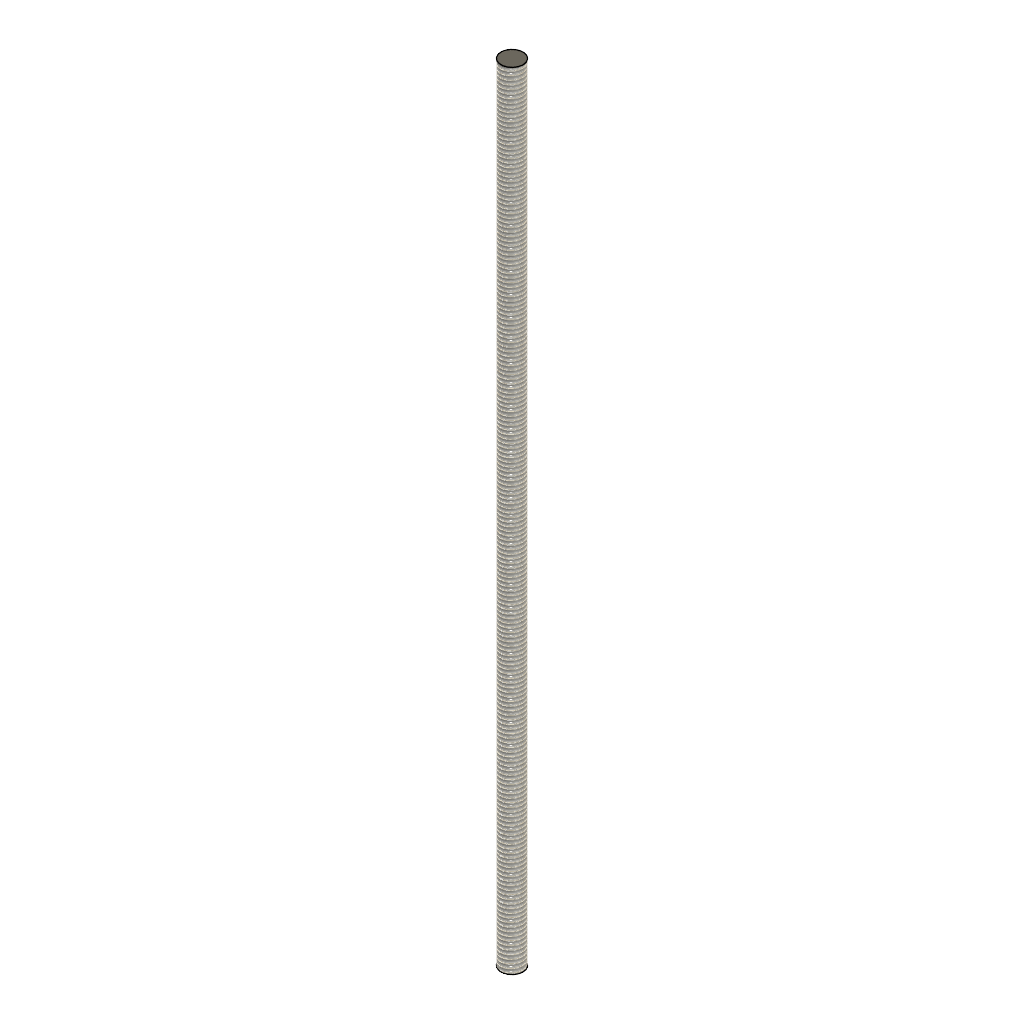
ROBOT_BALANCIN (Autodesk Fusion 360 archive; units mm, degrees)
design "M4_SIN_FIN"
Autodesk Fusion 360 part; units mm, degrees
(part 1 of 2)
sketch "Boceto1" plane through (0, 0, 0) normal (0, 0, 1) x (1, 0, 0)
  circle A0 centre (0, 0) radius 2
  dimension "d1" = 4
  constraint coincident A0.centre origin
  measures "d1" diameter of A0
extrude "Extruir1" add sketch "Boceto1" along normal blind 138
thread "Rosca1" "ISO Metric profile 4.0 M4x0.7 M4x0.7 6g" major diameter 3.908 minor diameter 3.111 pitch 0.7 angle 60 resizes the face on face at (1.9975, -0.0997, 92)
equation "d2 = 150 mm - 12 mm"

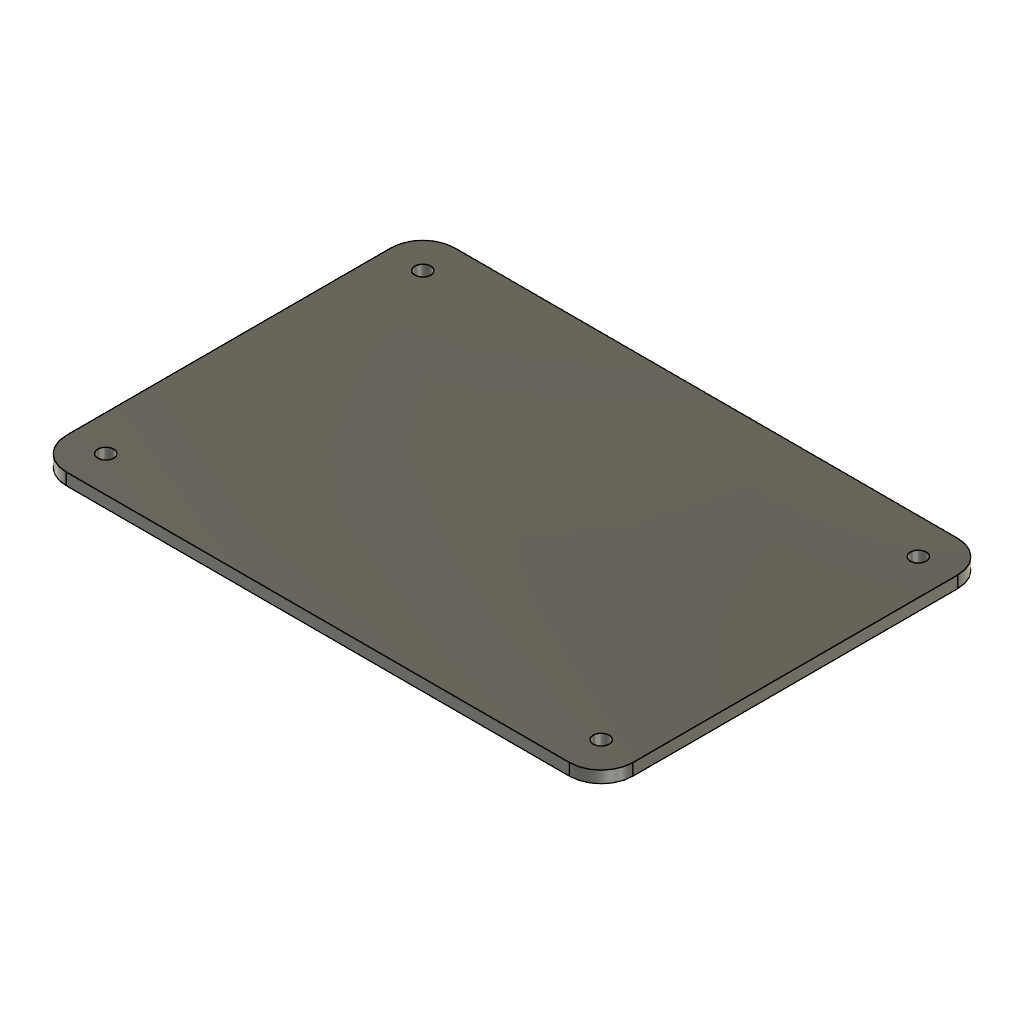
design "TAPA_BALANCIN"
Autodesk Fusion 360 part; units mm, degrees
sketch "Boceto1" plane through (0, 0, 0) normal (0, 0, 1) x (1, 0, 0)
  line L0 (71.5, 0) -> (-71.5, 0)
  line L1 (0, -49) -> (0, 49)
  line L2 (-71.5, 49) -> (71.5, 49)
  line L3 (71.5, 49) -> (71.5, -49)
  line L4 (71.5, -49) -> (-71.5, -49)
  line L5 (-71.5, -49) -> (-71.5, 49)
  line L6 (-71.5, 49) -> (71.5, -49) construction
  line L7 (71.5, 49) -> (-71.5, -49) construction
  dimension "d1" = 143
  dimension "d2" = 98
  constraint midpoint L0 origin
  constraint horizontal L0
  constraint midpoint L1 origin
  constraint perpendicular L0 L1
  constraint horizontal L2
  constraint perpendicular L2 L3
  constraint parallel L2 L4
  constraint parallel L3 L5
  constraint coincident L6 origin
  constraint coincident L7 origin
  measures "d1" distance of L0.start L0.end
  measures "d2" distance of L1.start L1.end
extrude "Extruir1" add sketch "Boceto1" along normal blind 3
sketch "Boceto2" plane through (0, 0, 3) normal (0, 0, 1) x (-1, 0, 0)
  line L0 (71.5, 49) -> (-71.5, 49)
  line L1 (-71.5, 49) -> (-71.5, -49)
  line L2 (-71.5, -49) -> (71.5, -49)
  line L3 (71.5, -49) -> (71.5, 49)
  line L4 (71.5, -49) -> (62.5, -49)
  line L5 (62.5, -49) -> (62.5, -40)
  line L6 (71.5, 49) -> (62.5, 49)
  line L7 (62.5, 49) -> (62.5, 40)
  line L8 (-71.5, 49) -> (-71.5, 40)
  line L9 (-71.5, 40) -> (-62.5, 40)
  line L10 (-71.5, -49) -> (-62.5, -49)
  line L11 (-62.5, -49) -> (-62.5, -40)
  circle A0 centre (62.5, -40) radius 2
  circle A1 centre (62.5, 40) radius 2
  circle A2 centre (-62.5, -40) radius 2
  circle A3 centre (-62.5, 40) radius 2
  dimension "d7" = 9
  dimension "d8" = 9
  dimension "d9" = 9
  dimension "d10" = 9
  dimension "d11" = 9
  dimension "d12" = 9
  dimension "d13" = 9
  dimension "d14" = 9
  dimension "d15" = 4
  dimension "d16" = 4
  dimension "d17" = 4
  dimension "d18" = 4
  constraint coincident L2.end L3.start
  constraint perpendicular L3 L4
  constraint perpendicular L2 L5
  constraint coincident L0.start L3.end
  constraint perpendicular L3 L6
  constraint perpendicular L6 L7
  constraint coincident L0.end L1.start
  constraint perpendicular L0 L8
  constraint perpendicular L1 L9
  constraint coincident L1.end L2.start
  constraint perpendicular L1 L10
  constraint perpendicular L2 L11
  constraint coincident L5.end A0.centre
  constraint coincident L7.end A1.centre
  constraint coincident L11.end A2.centre
  constraint coincident L9.end A3.centre
  measures "d7" distance of L2.end L4.end
  measures "d8" distance of L4.end L5.end
  measures "d9" distance of L0.start L6.end
  measures "d10" distance of L6.end L7.end
  measures "d11" distance of L0.end L8.end
  measures "d12" distance of L8.end L9.end
  measures "d13" distance of L1.end L10.end
  measures "d14" distance of L10.end L11.end
  measures "d15" diameter of A0
  measures "d16" diameter of A1
  measures "d17" diameter of A2
  measures "d18" diameter of A3
extrude "Extruir2" cut sketch "Boceto2" against normal blind 3 contours A0 | A1 | A2 | A3
fillet "Empalme2" radius 8 4 edges at (-71.5, -49, 1.5) (-71.5, 49, 1.5) (71.5, -49, 1.5) (71.5, 49, 1.5)

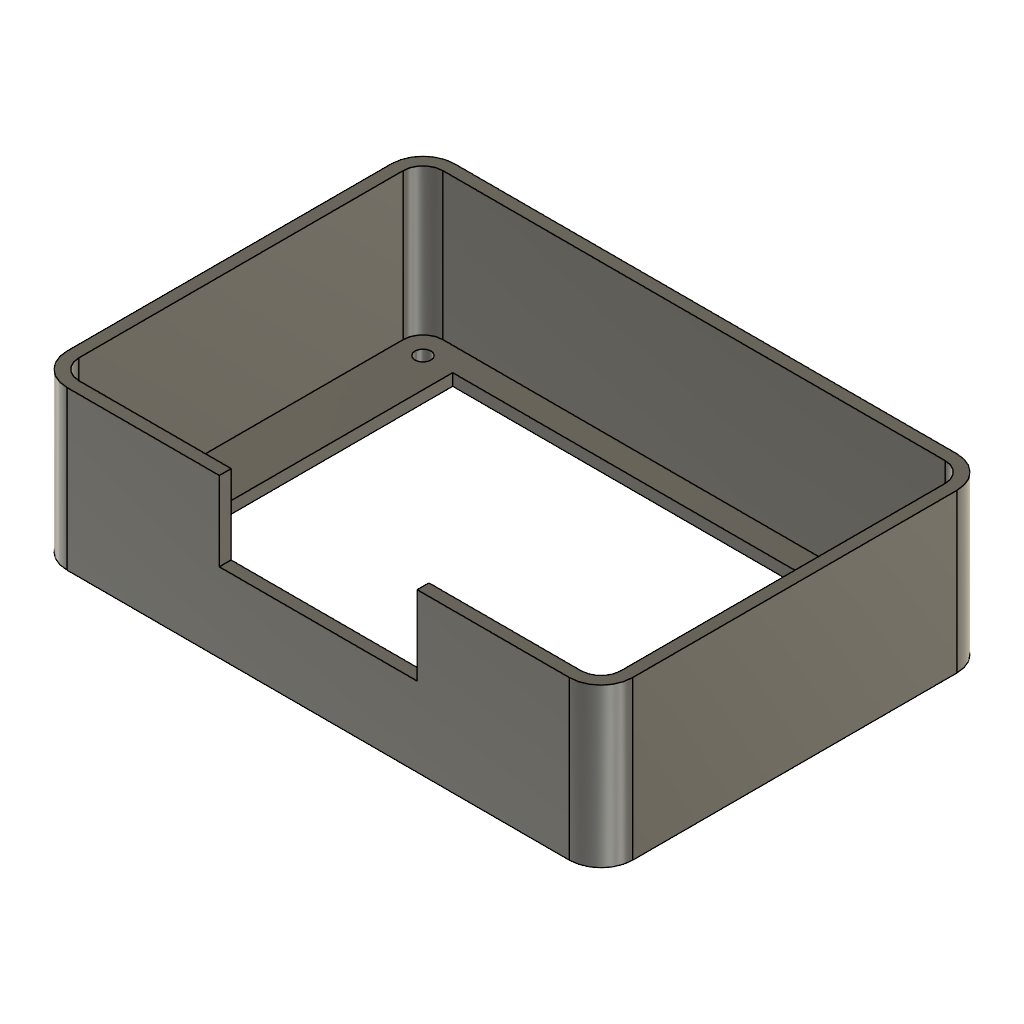
design "BASE_PCB"
Autodesk Fusion 360 part; units mm, degrees
sketch "Boceto1" plane through (0, 0, 0) normal (0, 0, 1) x (1, 0, 0)
  line L0 (-68.5, 46) -> (68.5, 46)
  line L1 (68.5, 46) -> (68.5, -46)
  line L2 (68.5, -46) -> (-68.5, -46)
  line L3 (-68.5, -46) -> (-68.5, 46)
  line L4 (-68.5, 46) -> (68.5, -46) construction
  line L5 (68.5, 46) -> (-68.5, -46) construction
  dimension "d1" = 137
  dimension "d2" = 92
  constraint horizontal L0
  constraint perpendicular L0 L1
  constraint parallel L0 L2
  constraint parallel L1 L3
  constraint coincident L4 origin
  constraint coincident L5 origin
  measures "d1" distance of L1.end L2.end
extrude "Extruir1" add sketch "Boceto1" along normal blind 3 makes body 1
sketch "Boceto2" plane through (0, 0, 3) normal (0, 0, 1) x (-1, 0, 0)
  line L0 (68.5, 46) -> (-68.5, 46)
  line L1 (-68.5, 46) -> (-68.5, -46)
  line L2 (-68.5, -46) -> (68.5, -46)
  line L3 (68.5, -46) -> (68.5, 46)
  line L4 (68.5, -46) -> (62.5, -46)
  line L5 (62.5, -46) -> (62.5, -40)
  line L6 (-68.5, -46) -> (-62.5, -46)
  line L7 (-62.5, -46) -> (-62.5, -40)
  line L8 (68.5, 46) -> (62.5, 46)
  line L9 (62.5, 46) -> (62.5, 40)
  line L10 (-68.5, 46) -> (-68.5, 40)
  line L11 (-68.5, 40) -> (-62.5, 40)
  circle A0 centre (62.5, -40) radius 2
  circle A1 centre (62.5, 40) radius 2
  circle A2 centre (-62.5, -40) radius 2
  circle A3 centre (-62.5, 40) radius 2
  dimension "d5" = 6
  dimension "d6" = 6
  dimension "d7" = 6
  dimension "d8" = 6
  dimension "d9" = 6
  dimension "d10" = 6
  dimension "d11" = 6
  dimension "d12" = 6
  dimension "d13" = 4
  dimension "d14" = 4
  dimension "d15" = 4
  dimension "d16" = 4
  constraint coincident L2.end L3.start
  constraint perpendicular L3 L4
  constraint perpendicular L4 L5
  constraint coincident L1.end L2.start
  constraint perpendicular L1 L6
  constraint perpendicular L6 L7
  constraint coincident L0.start L3.end
  constraint perpendicular L3 L8
  constraint perpendicular L8 L9
  constraint coincident L0.end L1.start
  constraint perpendicular L0 L10
  constraint perpendicular L1 L11
  constraint coincident L5.end A0.centre
  constraint coincident L9.end A1.centre
  constraint coincident L7.end A2.centre
  constraint coincident L11.end A3.centre
  measures "d13" diameter of A0
  measures "d14" diameter of A1
  measures "d15" diameter of A2
  measures "d16" diameter of A3
extrude "Extruir2" cut sketch "Boceto2" against normal blind 3 contours A0 | A1 | A2 | A3 bodies 1
fillet "Empalme1" radius 5 4 edges at (-68.5, -46, 1.5) (68.5, -46, 1.5) (68.5, 46, 1.5) (-68.5, 46, 1.5) on bodies 1
sketch "Boceto3" plane through (0, 0, 3) normal (0, 0, 1) x (-1, 0, 0)
  circle A0 centre (62.5, -40) radius 2
  circle A1 centre (-62.5, -40) radius 2
  circle A2 centre (62.5, 40) radius 2
  circle A3 centre (-62.5, 40) radius 2
  arc A4 (63.5, -46) -> (68.5, -41) centre (63.5, -41) ccw
  line L0 (68.5, -41) -> (68.5, 41)
  arc A5 (68.5, 41) -> (63.5, 46) centre (63.5, 41) ccw
  line L1 (63.5, 46) -> (-63.5, 46)
  arc A6 (-63.5, 46) -> (-68.5, 41) centre (-63.5, 41) ccw
  line L2 (-68.5, 41) -> (-68.5, -41)
  arc A7 (-68.5, -41) -> (-63.5, -46) centre (-63.5, -41) ccw
  line L3 (-63.5, -46) -> (63.5, -46)
  line L4 (-71.5, 41) -> (-71.5, -41)
  arc A8 (-71.5, -41) -> (-63.5, -49) centre (-63.5, -41) ccw
  line L5 (-63.5, -49) -> (63.5, -49)
  arc A9 (63.5, -49) -> (71.5, -41) centre (63.5, -41) ccw
  line L6 (71.5, -41) -> (71.5, 41)
  arc A10 (71.5, 41) -> (63.5, 49) centre (63.5, 41) ccw
  line L7 (63.5, 49) -> (-63.5, 49)
  arc A11 (-63.5, 49) -> (-71.5, 41) centre (-63.5, 41) ccw
  dimension "d21" = 3
extrude "Extruir3" add sketch "Boceto3" along normal blind 37 and the other way blind 3 separate body contours L4 A8 L5 A9 L6 A10 L7 A11 makes body 2
sketch "Boceto5" plane through (0, 0, 0) normal (0, 0, -1) x (1, 0, 0)
  arc A0 (-68.5, -41) -> (-63.5, -46) centre (-63.5, -41) ccw
  line L0 (-63.5, -46) -> (63.5, -46)
  arc A1 (63.5, -46) -> (68.5, -41) centre (63.5, -41) ccw
  line L1 (68.5, -41) -> (68.5, 41)
  arc A2 (68.5, 41) -> (63.5, 46) centre (63.5, 41) ccw
  line L2 (63.5, 46) -> (-63.5, 46)
  arc A3 (-63.5, 46) -> (-68.5, 41) centre (-63.5, 41) ccw
  line L3 (-68.5, 41) -> (-68.5, -41)
  circle A4 centre (-62.5, -40) radius 2
  circle A5 centre (62.5, -40) radius 2
  circle A6 centre (-62.5, 40) radius 2
  circle A7 centre (62.5, 40) radius 2
  line L4 (55, 40) -> (-55, 40)
  line L5 (-55, 40) -> (-55, -40)
  line L6 (-55, -40) -> (55, -40)
  line L7 (55, -40) -> (55, 40)
  line L8 (55, 40) -> (-55, -40) construction
  line L9 (-55, 40) -> (55, -40) construction
  dimension "d32" = 110
  dimension "d33" = 80
  constraint horizontal L4
  constraint perpendicular L4 L5
  constraint parallel L4 L6
  constraint parallel L5 L7
  constraint coincident L8 origin
  constraint coincident L9 origin
  measures "d32" distance of L5.end L6.end
  measures "d33" distance of L4.end L5.end
extrude "Extruir5" cut sketch "Boceto5" against normal blind 3 contours L4 L5 L6 L7 bodies 1
sketch "Boceto6" plane through (0, -49, 0) normal (0, -1, 0) x (1, 0, 0)
  line L0 (63.5, 0) -> (63.5, 40)
  line L1 (63.5, 40) -> (-63.5, 40)
  line L2 (-63.5, 40) -> (-63.5, 0)
  line L3 (-63.5, 0) -> (63.5, 0)
  line L4 (25, 40) -> (-25, 40)
  line L5 (-25, 40) -> (-25, 20)
  line L6 (-25, 20) -> (25, 20)
  line L7 (25, 20) -> (25, 40)
  point P0 (0, 40)
  dimension "d36" = 50
  constraint midpoint L4 P0
  constraint coincident L1 P0
  constraint perpendicular L0 L4
  constraint perpendicular L4 L5
  constraint perpendicular L5 L6
  constraint perpendicular L4 L7
  measures "d36" distance of L4.start L4.end
extrude "Extruir6" cut sketch "Boceto6" against normal blind 5 contours L1 L4 L5 L6 L7 bodies 2

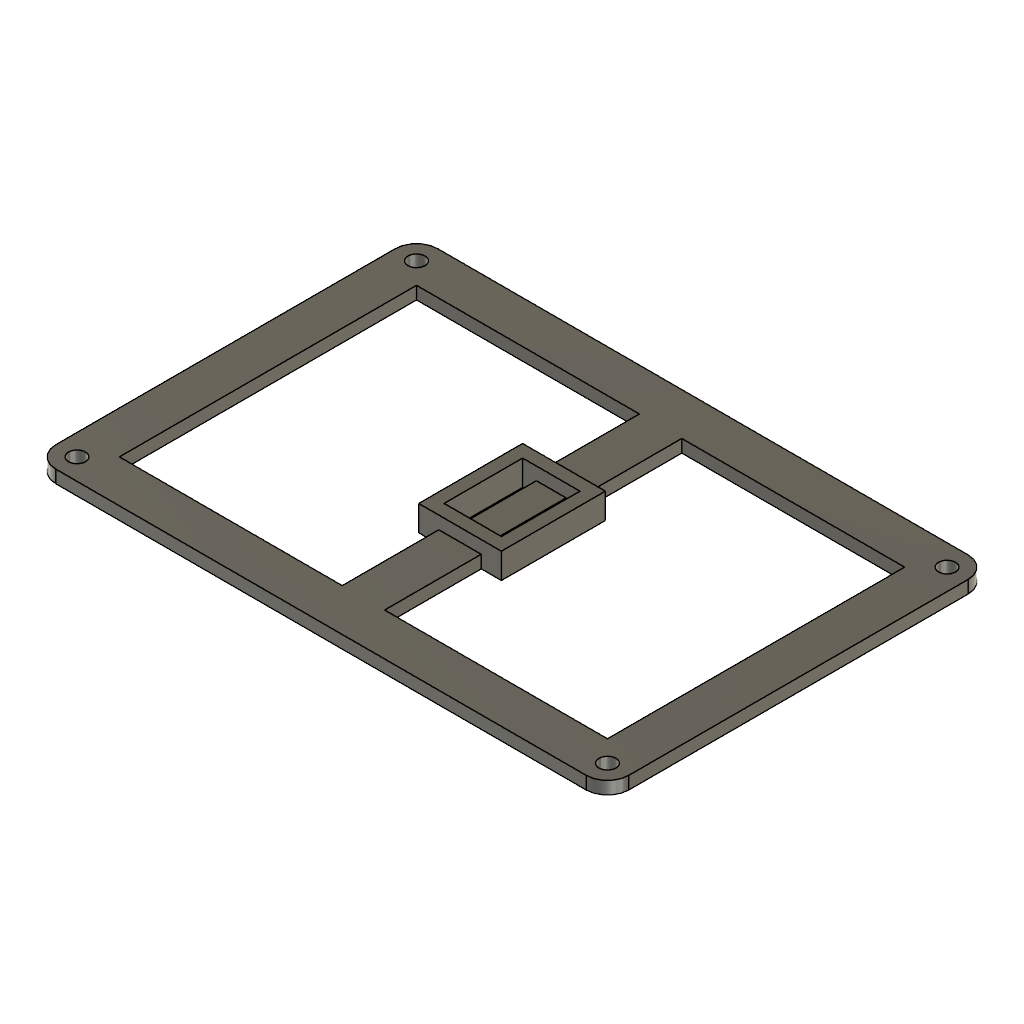
design "soporte_imu_inteligente"
Autodesk Fusion 360 part; units mm, degrees
sketch "Boceto1" plane through (0, 0, 0) normal (0, 0, 1) x (1, 0, 0)
  line L0 (-6.75, 9.25) -> (6.75, 9.25)
  line L1 (6.75, 9.25) -> (6.75, -9.25)
  line L2 (6.75, -9.25) -> (-6.75, -9.25)
  line L3 (-6.75, -9.25) -> (-6.75, 9.25)
  line L4 (-6.75, 9.25) -> (6.75, -9.25) construction
  line L5 (6.75, 9.25) -> (-6.75, -9.25) construction
  line L6 (9.75, -12.25) -> (-9.75, -12.25)
  line L7 (-9.75, -12.25) -> (-9.75, 12.25)
  line L8 (-9.75, 12.25) -> (9.75, 12.25)
  line L9 (9.75, 12.25) -> (9.75, -12.25)
  line L10 (6.75, 0) -> (3.75, 0) construction
  line L11 (-6.75, 0) -> (-3.75, 0) construction
  line L12 (3.5, 0) -> (-3.5, 0)
  line L13 (-3.5, -9.25) -> (-3.5, 9.25)
  line L14 (3.5, -9.25) -> (3.5, 9.25)
  dimension "d1" = 13.5
  dimension "d2" = 18.5
  dimension "d3" = -3
  dimension "d4" = 3
  dimension "d5" = 3
  dimension "d6" = 7
  constraint horizontal L0
  constraint perpendicular L0 L1
  constraint parallel L0 L2
  constraint parallel L1 L3
  constraint coincident L4 origin
  constraint coincident L5 origin
  constraint midpoint L1 L10.start
  constraint perpendicular L1 L10
  constraint midpoint L3 L11.start
  constraint perpendicular L3 L11
  constraint midpoint L12 origin
  constraint parallel L11 L12
  constraint midpoint L12.end L13
  constraint coincident L0 L13.end
  constraint perpendicular L0 L13
  constraint midpoint L12.start L14
  constraint coincident L0 L14.end
  constraint perpendicular L0 L14
  measures "d1" distance of L1.end L2.end
  measures "d2" distance of L0.end L1.end
  measures "d4" distance of L10.start L10.end
  measures "d5" distance of L11.start L11.end
  measures "d6" distance of L12.start L12.end
extrude "Extruir1" add sketch "Boceto1" along normal blind 6
extrude "Extruir2" add sketch "Boceto1" along normal blind 3 contours L0 L12 L13 L14 | L2 L12 L13 L14
sketch "Boceto2" plane through (0, 0, 0) normal (0, 0, -1) x (1, 0, 0)
  line L0 (-3.5, -9.25) -> (-6.75, -9.25)
  line L1 (-6.75, -9.25) -> (-6.75, 9.25)
  line L2 (-6.75, 9.25) -> (-3.5, 9.25)
  line L3 (-3.5, 9.25) -> (-3.5, -9.25)
  line L4 (3.5, -9.25) -> (3.5, 9.25)
  line L5 (3.5, 9.25) -> (6.75, 9.25)
  line L6 (6.75, 9.25) -> (6.75, -9.25)
  line L7 (6.75, -9.25) -> (3.5, -9.25)
  line L8 (-9.75, -12.25) -> (9.75, -12.25)
  line L9 (9.75, -12.25) -> (9.75, 12.25)
  line L10 (9.75, 12.25) -> (-9.75, 12.25)
  line L11 (-9.75, 12.25) -> (-9.75, -12.25)
  line L12 (-67.5, 45) -> (67.5, 45)
  line L13 (67.5, 45) -> (67.5, -45)
  line L14 (67.5, -45) -> (-67.5, -45)
  line L15 (-67.5, -45) -> (-67.5, 45)
  line L16 (-67.5, 45) -> (67.5, -45) construction
  line L17 (67.5, 45) -> (-67.5, -45) construction
  line L18 (-67.5, 45) -> (-62.5, 45)
  line L19 (-62.5, 45) -> (-62.5, 40)
  line L20 (-67.5, -45) -> (-62.5, -45)
  line L21 (-62.5, -45) -> (-62.5, -40)
  line L22 (67.5, -45) -> (62.5, -45)
  line L23 (62.5, -45) -> (62.5, -40)
  line L24 (67.5, 45) -> (62.5, 45)
  line L25 (62.5, 45) -> (62.5, 40)
  circle A0 centre (-62.5, 40) radius 2
  circle A1 centre (-62.5, -40) radius 2
  circle A2 centre (62.5, -40) radius 2
  circle A3 centre (62.5, 40) radius 2
  line L26 (0, -12.25) -> (0, -40)
  line L27 (0, 12.25) -> (0, 40)
  line L28 (-62.5, -40) -> (-62.5, 40) construction
  line L29 (62.5, -40) -> (62.5, 40) construction
  circle A4 centre (-62.5, 40) radius 5
  circle A5 centre (62.5, 40) radius 5
  circle A6 centre (-62.5, -40) radius 5
  circle A7 centre (62.5, -40) radius 5
  line L30 (5, -40) -> (-5, -40)
  line L31 (5, 40) -> (-5, 40)
  line L32 (-5, 40) -> (-5, 12.25)
  line L33 (5, 40) -> (5, 12.25)
  line L34 (-5, -40) -> (-5, -12.25)
  line L35 (5, -40) -> (5, -12.25)
  line L36 (-62.5, -45) -> (62.5, -45)
  arc A8 (62.5, -45) -> (62.5, -35) centre (62.5, -40) ccw
  line L37 (62.5, -35) -> (-62.5, -35)
  arc A9 (-62.5, -35) -> (-62.5, -45) centre (-62.5, -40) ccw
  line L38 (-62.5, -40) -> (62.5, -40) construction
  line L39 (-62.5, 35) -> (62.5, 35)
  arc A10 (62.5, 35) -> (62.5, 45) centre (62.5, 40) ccw
  line L40 (62.5, 45) -> (-62.5, 45)
  arc A11 (-62.5, 45) -> (-62.5, 35) centre (-62.5, 40) ccw
  line L41 (-62.5, 40) -> (62.5, 40) construction
  line L42 (-57.5, -40) -> (-57.5, 40)
  arc A12 (-57.5, 40) -> (-67.5, 40) centre (-62.5, 40) ccw
  line L43 (-67.5, 40) -> (-67.5, -40)
  arc A13 (-67.5, -40) -> (-57.5, -40) centre (-62.5, -40) ccw
  line L44 (-62.5, -40) -> (-62.5, 40) construction
  line L45 (67.5, -40) -> (67.5, 40)
  arc A14 (67.5, 40) -> (57.5, 40) centre (62.5, 40) ccw
  line L46 (57.5, 40) -> (57.5, -40)
  arc A15 (57.5, -40) -> (67.5, -40) centre (62.5, -40) ccw
  line L47 (62.5, -40) -> (62.5, 40) construction
  dimension "d11" = 135
  dimension "d12" = 90
  dimension "d13" = 5
  dimension "d14" = 5
  dimension "d15" = 5
  dimension "d16" = 5
  dimension "d17" = 5
  dimension "d18" = 5
  dimension "d19" = 5
  dimension "d20" = 5
  dimension "d21" = 4
  dimension "d22" = 4
  dimension "d23" = 4
  dimension "d24" = 4
  dimension "d25" = 10
  dimension "d26" = 10
  dimension "d27" = 10
  dimension "d28" = 10
  dimension "d29" = 10
  dimension "d30" = 10
  dimension "d31" = 10
  dimension "d32" = 10
  constraint horizontal L12
  constraint perpendicular L12 L13
  constraint parallel L12 L14
  constraint parallel L13 L15
  constraint coincident L16 origin
  constraint coincident L17 origin
  constraint perpendicular L15 L18
  constraint perpendicular L18 L19
  constraint perpendicular L15 L20
  constraint perpendicular L20 L21
  constraint perpendicular L13 L22
  constraint perpendicular L22 L23
  constraint perpendicular L13 L24
  constraint perpendicular L12 L25
  constraint coincident L19.end A0.centre
  constraint coincident L21.end A1.centre
  constraint coincident L23.end A2.centre
  constraint coincident L25.end A3.centre
  constraint midpoint L8 L26.start
  constraint perpendicular L14 L26
  constraint midpoint L10 L27.start
  constraint perpendicular L10 L27
  constraint concentric A0 A4
  constraint concentric A3 A5
  constraint concentric A1 A6
  constraint concentric A2 A7
  constraint midpoint L26.end L30
  constraint perpendicular L26 L30
  constraint midpoint L27.end L31
  constraint perpendicular L27 L31
  constraint coincident L10 L32.end
  constraint perpendicular L2 L32
  constraint coincident L10 L33.end
  constraint perpendicular L10 L33
  constraint coincident L8 L34.end
  constraint perpendicular L8 L34
  constraint coincident L8 L35.end
  constraint perpendicular L8 L35
  constraint tangent L36 A8
  constraint tangent A8 L37
  constraint parallel L36 L37
  constraint tangent L37 A9
  constraint tangent L36 A9
  constraint perpendicular L23 L38
  constraint tangent L39 A10
  constraint tangent A10 L40
  constraint parallel L39 L40
  constraint tangent L40 A11
  constraint tangent L39 A11
  constraint perpendicular L29 L41
  constraint tangent L42 A12
  constraint tangent A12 L43
  constraint parallel L42 L43
  constraint tangent L43 A13
  constraint tangent L42 A13
  constraint perpendicular L41 L44
  constraint tangent L45 A14
  constraint tangent A14 L46
  constraint parallel L45 L46
  constraint tangent L46 A15
  constraint tangent L45 A15
  constraint perpendicular L41 L47
  measures "d29" distance of L30.start L30.end
  measures "d30" distance of L31.start L31.end
extrude "Extruir3" add sketch "Boceto2" against normal blind 3 contours L8 L26 L34 L37 | L8 L26 L35 L37 | L26 L30 L34 L37 | L14 A6 A7 L30 L34 L35 L36 L37 L42 A13 L46 A15 | L10 L27 L32 L39 | L26 L30 L35 L37 | A6 L37 L42 | L15 A4 A6 L37 A9 L39 A11 L42 L43 | L10 L27 L33 L39 | L12 A4 A5 L31 L32 L33 L39 L40 L42 A12 A14 L46 | L27 L31 L32 L39 | A6 A9 A13 | A4 L39 L42 | L27 L31 L33 L39 | L13 A5 A7 A8 L37 L39 A10 L45 L46 | A7 L37 L46 | A4 A11 A12 | A7 A8 A15 | A5 L39 L46 | A5 A10 A14

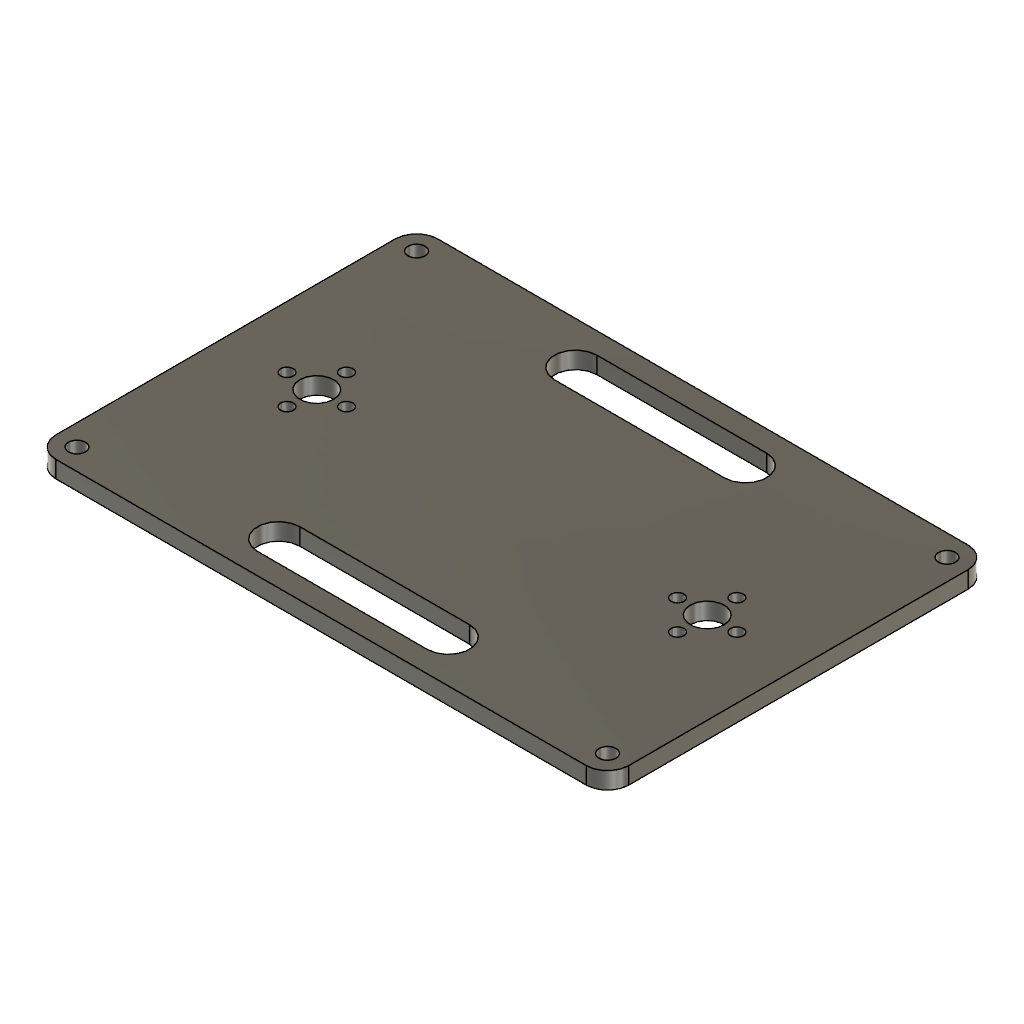
design "BASE_BALANCIN"
Autodesk Fusion 360 part; units mm, degrees
sketch "Boceto1" plane through (0, 0, 0) normal (0, 0, 1) x (1, 0, 0)
  line L0 (-67.5, 45) -> (67.5, 45)
  line L1 (67.5, 45) -> (67.5, -45)
  line L2 (67.5, -45) -> (-67.5, -45)
  line L3 (-67.5, -45) -> (-67.5, 45)
  line L4 (-67.5, 45) -> (67.5, -45) construction
  line L5 (67.5, 45) -> (-67.5, -45) construction
  dimension "d1" = 135
  dimension "d2" = 90
  constraint horizontal L0
  constraint perpendicular L0 L1
  constraint parallel L0 L2
  constraint parallel L1 L3
  constraint coincident L4 origin
  constraint coincident L5 origin
  measures "d1" distance of L1.end L2.end
extrude "Extruir1" add sketch "Boceto1" along normal blind 4
sketch "Boceto2" plane through (0, 0, 4) normal (0, 0, 1) x (-1, 0, 0)
  line L0 (67.5, 45) -> (-67.5, 45)
  line L1 (-67.5, 45) -> (-67.5, -45)
  line L2 (-67.5, -45) -> (67.5, -45)
  line L3 (67.5, -45) -> (67.5, 45)
  line L4 (67.5, -45) -> (67.5, -40)
  line L5 (67.5, -40) -> (62.5, -40)
  line L6 (67.5, 45) -> (62.5, 45)
  line L7 (62.5, 45) -> (62.5, 40)
  line L8 (-67.5, -45) -> (-62.5, -45)
  line L9 (-62.5, -45) -> (-62.5, -40)
  line L10 (-67.5, 45) -> (-67.5, 40)
  line L11 (-67.5, 40) -> (-62.5, 40)
  circle A0 centre (62.5, -40) radius 2
  circle A1 centre (62.5, 40) radius 2
  circle A2 centre (-62.5, -40) radius 2
  circle A3 centre (-62.5, 40) radius 2
  dimension "d5" = 5
  dimension "d6" = 5
  dimension "d7" = 135
  dimension "d8" = 90
  dimension "d9" = 5
  dimension "d10" = 5
  dimension "d11" = 5
  dimension "d12" = 5
  dimension "d13" = 5
  dimension "d14" = 5
  dimension "d15" = 4
  dimension "d16" = 4
  dimension "d17" = 4
  dimension "d18" = 4
  constraint coincident L2.end L3.start
  constraint perpendicular L2 L4
  constraint perpendicular L3 L5
  constraint coincident L0.start L3.end
  constraint perpendicular L3 L6
  constraint perpendicular L0 L7
  constraint coincident L1.end L2.start
  constraint perpendicular L1 L8
  constraint perpendicular L2 L9
  constraint coincident L0.end L1.start
  constraint perpendicular L0 L10
  constraint perpendicular L1 L11
  constraint coincident L5.end A0.centre
  constraint coincident L7.end A1.centre
  constraint coincident L9.end A2.centre
  constraint coincident L11.end A3.centre
  measures "d1" distance of L1.end L2.end
extrude "Extruir2" cut sketch "Boceto2" against normal blind 4 contours A0 | A1 | A2 | A3
fillet "Empalme1" radius 5 4 edges at (-67.5, -45, 2) (67.5, -45, 2) (67.5, 45, 2) (-67.5, 45, 2)
sketch "Boceto3" plane through (0, 0, 4) normal (0, 0, 1) x (-1, 0, 0)
  circle A0 centre (62.5, 40) radius 2
  circle A1 centre (-62.5, -40) radius 2
  circle A2 centre (62.5, -40) radius 2
  circle A3 centre (-62.5, 40) radius 2
  arc A4 (62.5, -45) -> (67.5, -40) centre (62.5, -40) ccw
  line L0 (67.5, -40) -> (67.5, 40)
  arc A5 (67.5, 40) -> (62.5, 45) centre (62.5, 40) ccw
  line L1 (62.5, 45) -> (-62.5, 45)
  arc A6 (-62.5, 45) -> (-67.5, 40) centre (-62.5, 40) ccw
  line L2 (-67.5, 40) -> (-67.5, -40)
  arc A7 (-67.5, -40) -> (-62.5, -45) centre (-62.5, -40) ccw
  line L3 (-62.5, -45) -> (62.5, -45)
  line L4 (-67.5, 0) -> (-46, 0)
  circle A8 centre (-46, 0) radius 4
  circle A9 centre (-46, 0) radius 7
  line L5 (-46, 0) -> (-46, -7) construction
  line L6 (-46, 0) -> (-39, 0) construction
  line L7 (-46, 0) -> (-46, 7) construction
  line L8 (-46, 0) -> (-53, 0) construction
  circle A10 centre (-46, -7) radius 1.5
  circle A11 centre (-39, 0) radius 1.5
  circle A12 centre (-46, 7) radius 1.5
  circle A13 centre (-53, 0) radius 1.5
  dimension "d23" = 21.5
  dimension "d24" = 8
  dimension "d25" = 14
  dimension "d26" = 3
  dimension "d27" = 3
  dimension "d28" = 3
  dimension "d29" = 3
  constraint midpoint L2 L4.start
  constraint perpendicular L2 L4
  constraint coincident L4.end A8.centre
  constraint concentric A8 A9
  constraint coincident A9 L5.end
  constraint perpendicular L4 L5
  constraint coincident A9 L6.end
  constraint perpendicular L5 L6
  constraint coincident A9 L7.end
  constraint perpendicular L6 L7
  constraint coincident L4 L8.end
  constraint coincident A9 L8.end
  constraint coincident L5.end A10.centre
  constraint coincident L6.end A11.centre
  constraint coincident L7.end A12.centre
  constraint coincident L8.end A13.centre
  measures "d23" distance of L4.start L4.end
  measures "d24" diameter of A8
  measures "d25" diameter of A9
  measures "d26" diameter of A10
  measures "d27" diameter of A11
  measures "d28" diameter of A12
  measures "d29" diameter of A13
extrude "Extruir3" cut sketch "Boceto3" against normal blind 4 contours L4 A9 A13 | L4 A9 A13 | L4 A9 A13 | L4 A9 A13 | A9 A12 | A9 A12 | A9 A10 | A9 A10 | A9 A11 | A9 A11 | A8
mirror "Simetría1" about plane through (0, 0, 0) normal (1, 0, 0) of "Extruir3"
sketch "Boceto4" plane through (0, 0, 4) normal (0, 0, 1) x (-1, 0, 0)
  circle A0 centre (46, 7) radius 1.5
  circle A1 centre (46, -7) radius 1.5
  circle A2 centre (39, 0) radius 1.5
  circle A3 centre (53, 0) radius 1.5
  circle A4 centre (46, 0) radius 4
  arc A5 (62.5, -45) -> (67.5, -40) centre (62.5, -40) ccw
  line L0 (67.5, -40) -> (67.5, 40)
  arc A6 (67.5, 40) -> (62.5, 45) centre (62.5, 40) ccw
  line L1 (62.5, 45) -> (-62.5, 45)
  arc A7 (-62.5, 45) -> (-67.5, 40) centre (-62.5, 40) ccw
  line L2 (-67.5, 40) -> (-67.5, -40)
  arc A8 (-67.5, -40) -> (-62.5, -45) centre (-62.5, -40) ccw
  line L3 (-62.5, -45) -> (62.5, -45)
  circle A9 centre (-62.5, 40) radius 2
  circle A10 centre (62.5, -40) radius 2
  circle A11 centre (-62.5, -40) radius 2
  circle A12 centre (62.5, 40) radius 2
  circle A13 centre (-46, 7) radius 1.5
  circle A14 centre (-46, -7) radius 1.5
  circle A15 centre (-53, 0) radius 1.5
  circle A16 centre (-39, 0) radius 1.5
  circle A17 centre (-46, 0) radius 4
  line L4 (0, 35) -> (0, -35)
  line L5 (-20, -35) -> (20, -35)
  line L6 (-20, 35) -> (20, 35)
  line L7 (20, -30) -> (-20, -30)
  arc A18 (-20, -30) -> (-20, -40) centre (-20, -35) ccw
  line L8 (-20, -40) -> (20, -40)
  arc A19 (20, -40) -> (20, -30) centre (20, -35) ccw
  line L9 (20, -35) -> (-20, -35) construction
  line L10 (20, 40) -> (-20, 40)
  arc A20 (-20, 40) -> (-20, 30) centre (-20, 35) ccw
  line L11 (-20, 30) -> (20, 30)
  arc A21 (20, 30) -> (20, 40) centre (20, 35) ccw
  line L12 (20, 35) -> (-20, 35) construction
  dimension "d34" = 70
  dimension "d35" = 40
  dimension "d36" = 40
  dimension "d37" = 10
  dimension "d38" = 10
  constraint midpoint L4 origin
  constraint vertical L4
  constraint midpoint L4.end L5
  constraint perpendicular L4 L5
  constraint midpoint L4.start L6
  constraint perpendicular L4 L6
  constraint tangent L7 A18
  constraint tangent A18 L8
  constraint parallel L7 L8
  constraint tangent L8 A19
  constraint tangent L7 A19
  constraint coincident L5.start A18.centre
  constraint perpendicular L4 L9
  constraint coincident L5.end A19.centre
  constraint tangent L10 A20
  constraint tangent A20 L11
  constraint parallel L10 L11
  constraint tangent L11 A21
  constraint tangent L10 A21
  constraint coincident L6.start A20.centre
  constraint perpendicular L4 L12
  constraint coincident L6.end A21.centre
  measures "d34" distance of L4.start L4.end
  measures "d35" distance of L5.start L5.end
  measures "d36" distance of L6.start L6.end
  measures "d37" diameter of A18
  measures "d38" diameter of A20
extrude "Extruir4" cut sketch "Boceto4" against normal blind 4 contours L7 A18 L8 A19 | L10 A20 L11 A21

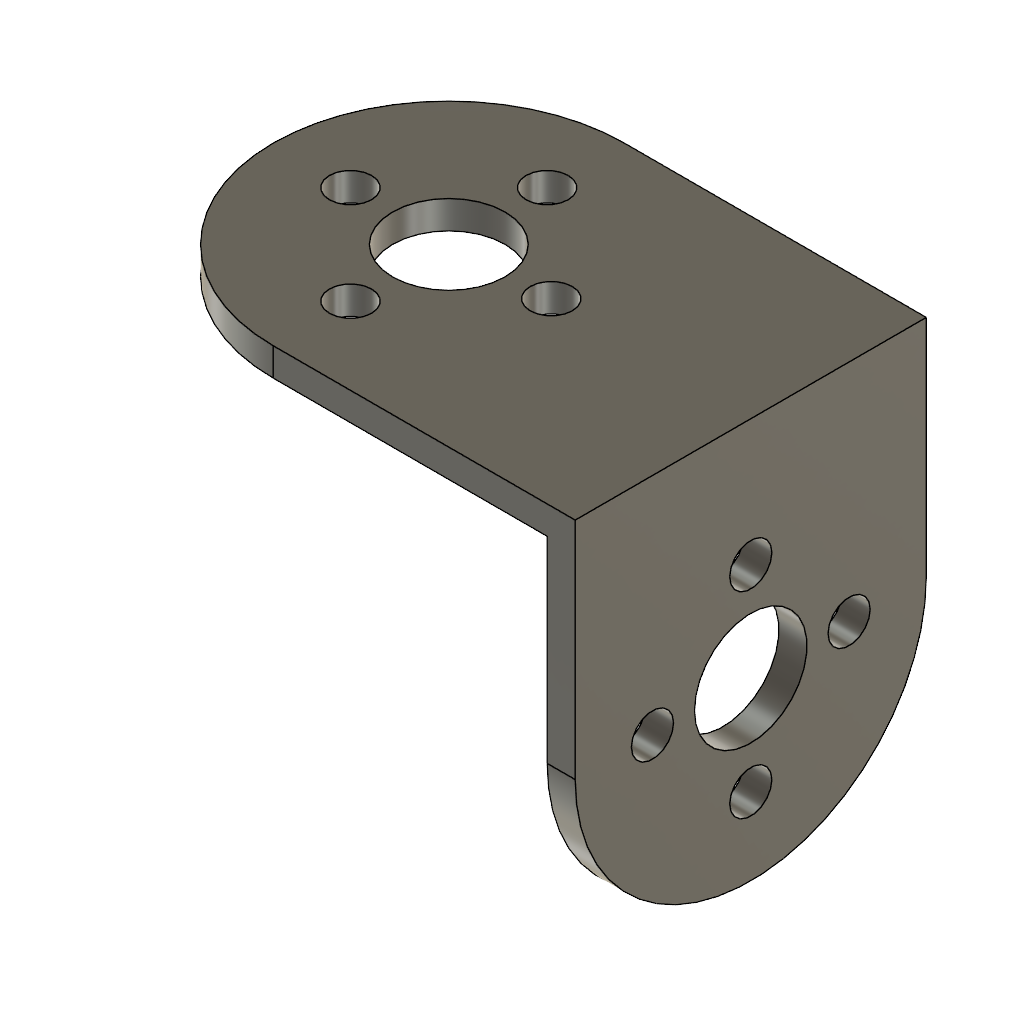
design "soporte_motor_12V_inteligente"
Autodesk Fusion 360 part; units mm, degrees
sketch "Boceto1" plane through (0, 0, 0) normal (0, 0, 1) x (1, 0, 0)
  line L0 (0, 12.5) -> (0, -12.5)
  arc A0 (0, 12.5) -> (0, -12.5) centre (0, 0) ccw
  line L1 (0, 12.5) -> (19.5, 12.5)
  line L2 (0, -12.5) -> (19.5, -12.5)
  line L3 (19.5, -12.5) -> (19.5, 12.5)
  circle A1 centre (0, 0) radius 4
  circle A2 centre (0, 0) radius 7 construction
  circle A3 centre (0, 7) radius 1.5
  circle A4 centre (-7, 0) radius 1.5
  circle A5 centre (0, -7) radius 1.5
  circle A6 centre (6.9935, 0.3006) radius 1.5
  dimension "d1" = 25
  dimension "d2" = 19.5
  dimension "d3" = 19.5
  dimension "d4" = 8
  dimension "d5" = 14
  dimension "d6" = 3
  dimension "d7" = 3
  dimension "d8" = 3
  dimension "d9" = 3
  constraint coincident A0.centre A1.centre
  constraint perpendicular L0 A0
  constraint perpendicular L0 L1
  constraint perpendicular L0 L2
  constraint concentric A0 A2
  constraint coincident A2 A3.centre
  constraint coincident L0 A3.centre
  constraint coincident A2 A4.centre
  constraint coincident A2 A5.centre
  constraint coincident L0 A5.centre
  constraint coincident A2 A6.centre
  measures "d1" diameter of A0
  measures "d2" distance of L0.start L1.end
  measures "d3" distance of L0.end L2.end
  measures "d4" diameter of A1
  measures "d5" diameter of A2
  measures "d6" diameter of A3
  measures "d7" diameter of A4
  measures "d8" diameter of A5
  measures "d9" diameter of A6
extrude "Extruir1" add sketch "Boceto1" along normal blind 2 contours L0 L1 L2 L3 A1 A3 A5 | L0 A0 A1 A3 A5
sketch "Boceto2" plane through (19.5, 0, 0) normal (1, 0, 0) x (0, 1, 0)
  line L0 (-12.5, 0) -> (12.5, 0)
  line L1 (12.5, 0) -> (12.5, 2)
  line L2 (12.5, 2) -> (-12.5, 2)
  line L3 (-12.5, 2) -> (-12.5, 0)
  line L4 (12.5, 0) -> (12.5, -14)
  line L5 (-12.5, 0) -> (-12.5, -14)
  circle A0 centre (0, -14) radius 4
  circle A1 centre (0, -14) radius 7 construction
  circle A2 centre (0, -7) radius 1.5
  circle A3 centre (-7, -14) radius 1.5
  circle A4 centre (0, -21) radius 1.5
  circle A5 centre (7, -14) radius 1.5
  circle A6 centre (0, -14) radius 12.5
  line L6 (-12.5, 2) -> (12.5, 2)
  line L7 (12.5, 2) -> (12.5, 0)
  line L8 (12.5, 0) -> (-12.5, 0)
  line L9 (-12.5, 0) -> (-12.5, 2)
  dimension "d12" = 14
  dimension "d13" = 14
  dimension "d14" = 8
  dimension "d15" = 14
  dimension "d16" = 3
  dimension "d17" = 3
  dimension "d18" = 3
  dimension "d19" = 3
  constraint coincident L0.end L1.start
  constraint perpendicular L0 L4
  constraint coincident L0.start L3.end
  constraint perpendicular L0 L5
  constraint concentric A0 A1
  constraint coincident A1 A2.centre
  constraint coincident A1 A3.centre
  constraint coincident A1 A4.centre
  constraint coincident A1 A5.centre
  constraint concentric A0 A6
  constraint coincident L5.end A6
  constraint horizontal L6
  constraint vertical L7
  constraint horizontal L8
  constraint vertical L9
  constraint coincident L2.end L3.start
  measures "d12" distance of L0.end L4.end
  measures "d13" distance of L0.start L5.end
  measures "d14" diameter of A0
  measures "d15" diameter of A1
  measures "d16" diameter of A2
  measures "d17" diameter of A3
  measures "d18" diameter of A4
  measures "d19" diameter of A5
extrude "Extruir2" add sketch "Boceto2" along normal blind 2
equation "d1 = ( 12.5 * 2 ) * 1 mm"

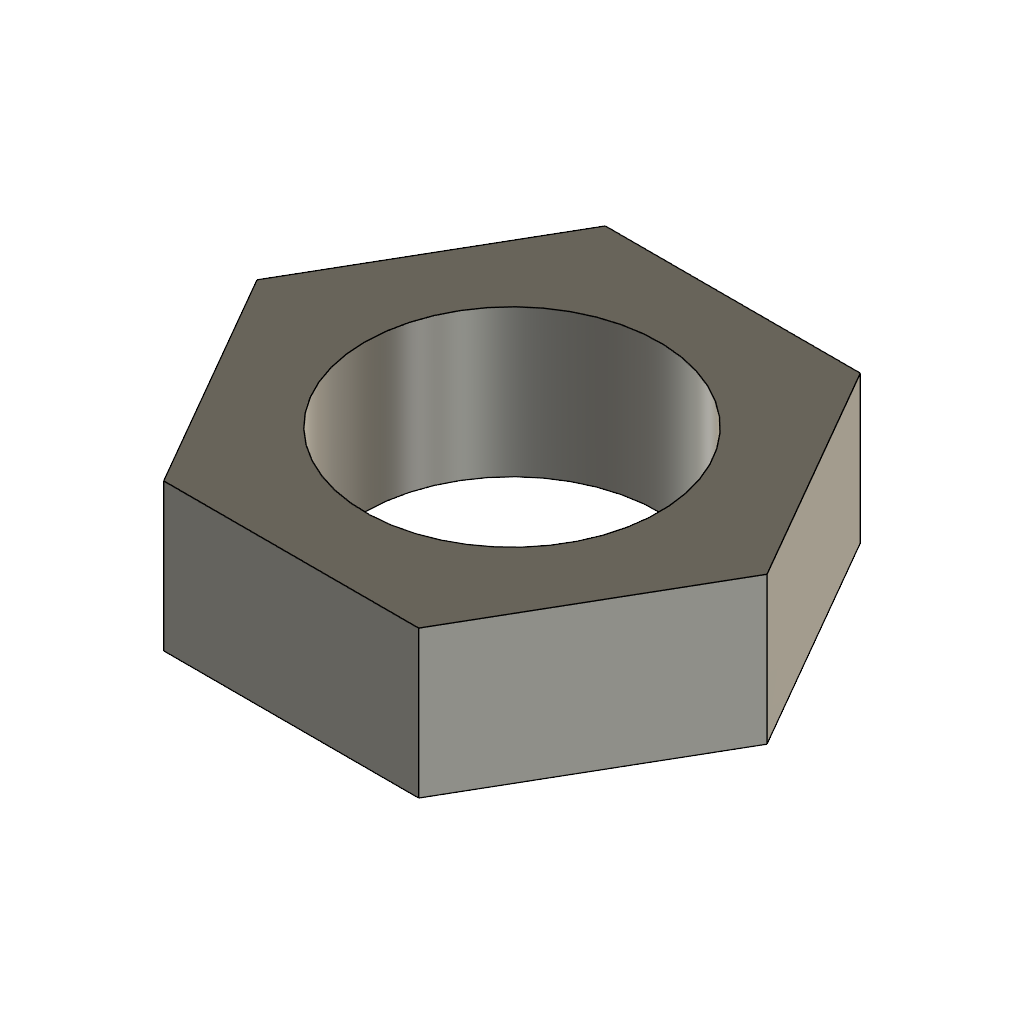
design "TUERCA_M4"
Autodesk Fusion 360 part; units mm, degrees
sketch "Boceto1" plane through (0, 0, 0) normal (0, 0, 1) x (1, 0, 0)
  circle A0 centre (0, 0) radius 2
  line L0 (-1.7321, 3) -> (-3.4641, 0)
  line L1 (-3.4641, 0) -> (-1.7321, -3)
  line L2 (-1.7321, -3) -> (1.7321, -3)
  line L3 (1.7321, -3) -> (3.4641, 0)
  line L4 (3.4641, 0) -> (1.7321, 3)
  line L5 (1.7321, 3) -> (-1.7321, 3)
  dimension "d1" = 4
  constraint coincident A0.centre origin
  measures "d1" diameter of A0
extrude "Extruir1" add sketch "Boceto1" along normal blind 2

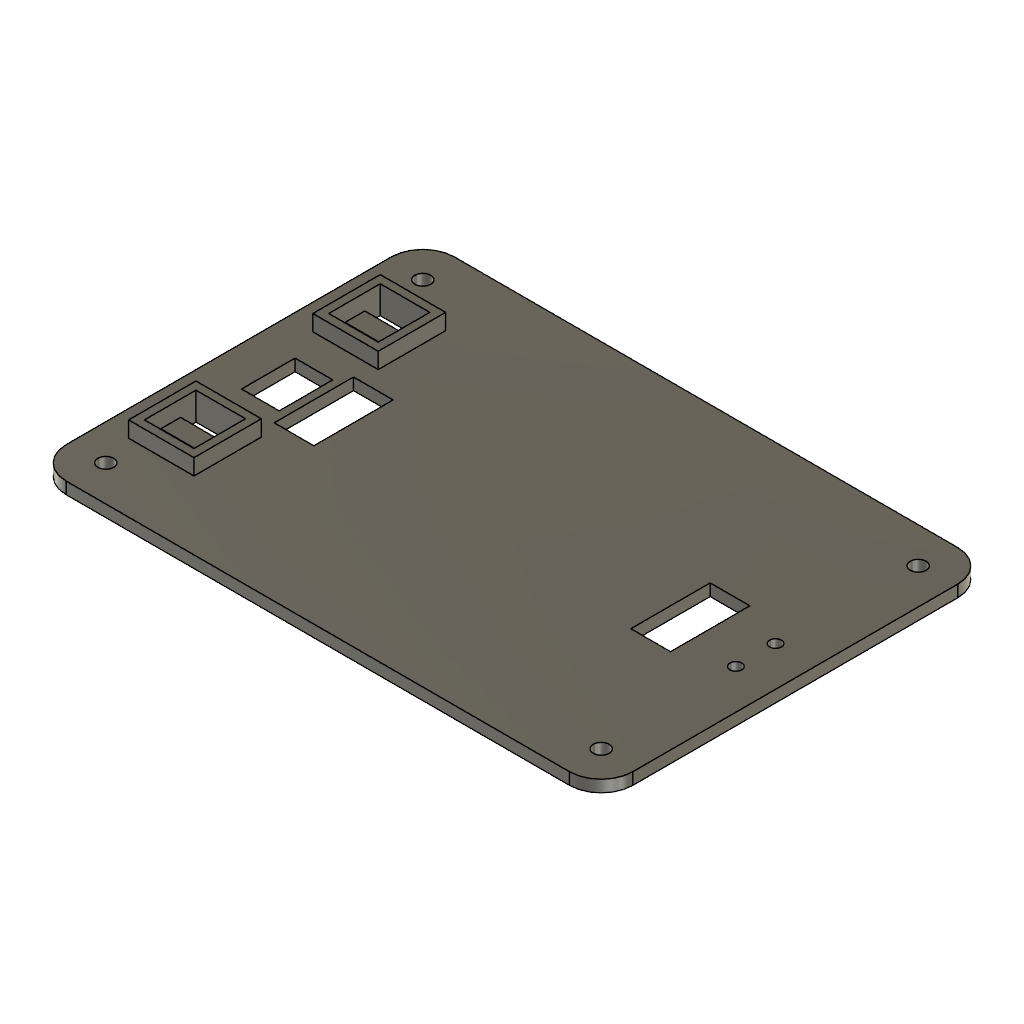
design "TAPA_BALANCIN_2"
Autodesk Fusion 360 part; units mm, degrees
sketch "Boceto1" plane through (0, 0, 0) normal (0, 0, 1) x (1, 0, 0)
  line L0 (71.5, 0) -> (-71.5, 0)
  line L1 (0, -49) -> (0, 49)
  line L2 (-71.5, 49) -> (71.5, 49)
  line L3 (71.5, 49) -> (71.5, -49)
  line L4 (71.5, -49) -> (-71.5, -49)
  line L5 (-71.5, -49) -> (-71.5, 49)
  line L6 (-71.5, 49) -> (71.5, -49) construction
  line L7 (71.5, 49) -> (-71.5, -49) construction
  dimension "d1" = 143
  dimension "d2" = 98
  constraint midpoint L0 origin
  constraint horizontal L0
  constraint midpoint L1 origin
  constraint perpendicular L0 L1
  constraint horizontal L2
  constraint perpendicular L2 L3
  constraint parallel L2 L4
  constraint parallel L3 L5
  constraint coincident L6 origin
  constraint coincident L7 origin
  measures "d1" distance of L0.start L0.end
  measures "d2" distance of L1.start L1.end
extrude "Extruir1" add sketch "Boceto1" along normal blind 3
sketch "Boceto2" plane through (0, 0, 3) normal (0, 0, 1) x (-1, 0, 0)
  line L0 (71.5, 49) -> (-71.5, 49)
  line L1 (-71.5, 49) -> (-71.5, -49)
  line L2 (-71.5, -49) -> (71.5, -49)
  line L3 (71.5, -49) -> (71.5, 49)
  line L4 (71.5, -49) -> (62.5, -49)
  line L5 (62.5, -49) -> (62.5, -40)
  line L6 (71.5, 49) -> (62.5, 49)
  line L7 (62.5, 49) -> (62.5, 40)
  line L8 (-71.5, 49) -> (-71.5, 40)
  line L9 (-71.5, 40) -> (-62.5, 40)
  line L10 (-71.5, -49) -> (-62.5, -49)
  line L11 (-62.5, -49) -> (-62.5, -40)
  circle A0 centre (62.5, -40) radius 2
  circle A1 centre (62.5, 40) radius 2
  circle A2 centre (-62.5, -40) radius 2
  circle A3 centre (-62.5, 40) radius 2
  dimension "d7" = 9
  dimension "d8" = 9
  dimension "d9" = 9
  dimension "d10" = 9
  dimension "d11" = 9
  dimension "d12" = 9
  dimension "d13" = 9
  dimension "d14" = 9
  dimension "d15" = 4
  dimension "d16" = 4
  dimension "d17" = 4
  dimension "d18" = 4
  constraint coincident L2.end L3.start
  constraint perpendicular L3 L4
  constraint perpendicular L2 L5
  constraint coincident L0.start L3.end
  constraint perpendicular L3 L6
  constraint perpendicular L6 L7
  constraint coincident L0.end L1.start
  constraint perpendicular L0 L8
  constraint perpendicular L1 L9
  constraint coincident L1.end L2.start
  constraint perpendicular L1 L10
  constraint perpendicular L2 L11
  constraint coincident L5.end A0.centre
  constraint coincident L7.end A1.centre
  constraint coincident L11.end A2.centre
  constraint coincident L9.end A3.centre
  measures "d7" distance of L2.end L4.end
  measures "d8" distance of L4.end L5.end
  measures "d9" distance of L0.start L6.end
  measures "d10" distance of L6.end L7.end
  measures "d11" distance of L0.end L8.end
  measures "d12" distance of L8.end L9.end
  measures "d13" distance of L1.end L10.end
  measures "d14" distance of L10.end L11.end
  measures "d15" diameter of A0
  measures "d16" diameter of A1
  measures "d17" diameter of A2
  measures "d18" diameter of A3
extrude "Extruir2" cut sketch "Boceto2" against normal blind 3 contours A0 | A1 | A2 | A3
fillet "Empalme2" radius 8 4 edges at (-71.5, -49, 1.5) (-71.5, 49, 1.5) (71.5, -49, 1.5) (71.5, 49, 1.5)
sketch "Boceto3" plane through (0, 0, 3) normal (0, 0, 1) x (-1, 0, 0)
  circle A0 centre (62.5, 40) radius 2
  circle A1 centre (-62.5, -40) radius 2
  circle A2 centre (62.5, -40) radius 2
  circle A3 centre (-62.5, 40) radius 2
  arc A4 (-71.5, -41) -> (-63.5, -49) centre (-63.5, -41) ccw
  line L0 (-63.5, -49) -> (63.5, -49)
  arc A5 (63.5, -49) -> (71.5, -41) centre (63.5, -41) ccw
  line L1 (71.5, -41) -> (71.5, 41)
  arc A6 (71.5, 41) -> (63.5, 49) centre (63.5, 41) ccw
  line L2 (63.5, 49) -> (-63.5, 49)
  arc A7 (-63.5, 49) -> (-71.5, 41) centre (-63.5, 41) ccw
  line L3 (-71.5, 41) -> (-71.5, -41)
  line L4 (-40, 0) -> (40, 0)
  line L5 (40, 10) -> (40, -10)
  line L6 (-40, 10) -> (-40, -10)
  line L7 (40, -10) -> (50, -10)
  line L8 (50, -10) -> (50, 10)
  line L9 (50, 10) -> (40, 10)
  line L10 (40, 10) -> (40, -10)
  line L11 (-40, -10) -> (-50, -10)
  line L12 (-50, -10) -> (-50, 10)
  line L13 (-50, 10) -> (-40, 10)
  line L14 (-40, 10) -> (-40, -10)
  dimension "d23" = 80
  dimension "d24" = 20
  dimension "d25" = 20
  dimension "d26" = 10
  dimension "d27" = 20
  dimension "d28" = 10
  dimension "d29" = 20
  constraint midpoint L4 origin
  constraint horizontal L4
  constraint midpoint L4.end L5
  constraint perpendicular L4 L5
  constraint midpoint L4.start L6
  constraint perpendicular L4 L6
  constraint horizontal L7
  constraint vertical L8
  constraint horizontal L9
  constraint vertical L10
  constraint horizontal L11
  constraint vertical L12
  constraint horizontal L13
  constraint vertical L14
  measures "d23" distance of L4.start L4.end
  measures "d24" distance of L5.start L5.end
  measures "d25" distance of L6.start L6.end
  measures "d26" distance of L5.end L7.end
  measures "d27" distance of L5.end L5.start
  measures "d28" distance of L6.end L11.end
  measures "d29" distance of L6.end L6.start
extrude "Extruir3" cut sketch "Boceto3" against normal blind 3 contours L5 L7 L8 L9 L10 | L6 L11 L12 L13 L14
sketch "Boceto4" plane through (0, 0, 3) normal (0, 0, 1) x (-1, 0, 0)
  line L0 (50, -10) -> (40, -10)
  line L1 (40, -10) -> (40, 10)
  line L2 (40, 10) -> (50, 10)
  line L3 (50, 10) -> (50, -10)
  line L4 (-50, -10) -> (-50, 10)
  line L5 (-50, 10) -> (-40, 10)
  line L6 (-40, 10) -> (-40, -10)
  line L7 (-40, -10) -> (-50, -10)
  circle A0 centre (62.5, 40) radius 2
  circle A1 centre (-62.5, -40) radius 2
  circle A2 centre (62.5, -40) radius 2
  circle A3 centre (-62.5, 40) radius 2
  arc A4 (-71.5, -41) -> (-63.5, -49) centre (-63.5, -41) ccw
  line L8 (-63.5, -49) -> (63.5, -49)
  arc A5 (63.5, -49) -> (71.5, -41) centre (63.5, -41) ccw
  line L9 (71.5, -41) -> (71.5, 41)
  arc A6 (71.5, 41) -> (63.5, 49) centre (63.5, 41) ccw
  line L10 (63.5, 49) -> (-63.5, 49)
  arc A7 (-63.5, 49) -> (-71.5, 41) centre (-63.5, 41) ccw
  line L11 (-71.5, 41) -> (-71.5, -41)
  line L12 (71.5, 0) -> (61.5, 0)
  line L13 (61.5, 6.75) -> (61.5, -6.75)
  line L14 (61.5, -6.75) -> (52, -6.75)
  line L15 (61.5, 6.75) -> (52, 6.75)
  line L16 (52, 6.75) -> (52, -6.75)
  dimension "d32" = 10
  dimension "d33" = 13.5
  dimension "d34" = 9.5
  dimension "d35" = 9.5
  constraint midpoint L9 L12.start
  constraint perpendicular L9 L12
  constraint midpoint L12.end L13
  constraint perpendicular L12 L13
  constraint perpendicular L13 L14
  constraint perpendicular L13 L15
  measures "d32" distance of L12.start L12.end
  measures "d33" distance of L13.start L13.end
  measures "d34" distance of L13.end L14.end
  measures "d35" distance of L13.start L15.end
extrude "Extruir4" cut sketch "Boceto4" against normal blind 3 contours L13 L14 L15 L16
sketch "Boceto5" plane through (0, 0, 3) normal (0, 0, 1) x (-1, 0, 0)
  line L0 (52, -6.75) -> (52, 6.75)
  line L1 (52, 6.75) -> (61.5, 6.75)
  line L2 (61.5, 6.75) -> (61.5, -6.75)
  line L3 (61.5, -6.75) -> (52, -6.75)
  line L4 (50, -10) -> (40, -10)
  line L5 (40, -10) -> (40, 10)
  line L6 (40, 10) -> (50, 10)
  line L7 (50, 10) -> (50, -10)
  line L8 (-50, -10) -> (-50, 10)
  line L9 (-50, 10) -> (-40, 10)
  line L10 (-40, 10) -> (-40, -10)
  line L11 (-40, -10) -> (-50, -10)
  circle A0 centre (62.5, 40) radius 2
  circle A1 centre (-62.5, -40) radius 2
  circle A2 centre (62.5, -40) radius 2
  circle A3 centre (-62.5, 40) radius 2
  arc A4 (-71.5, -41) -> (-63.5, -49) centre (-63.5, -41) ccw
  line L12 (-63.5, -49) -> (63.5, -49)
  arc A5 (63.5, -49) -> (71.5, -41) centre (63.5, -41) ccw
  line L13 (71.5, -41) -> (71.5, 41)
  arc A6 (71.5, 41) -> (63.5, 49) centre (63.5, 41) ccw
  line L14 (63.5, 49) -> (-63.5, 49)
  arc A7 (-63.5, 49) -> (-71.5, 41) centre (-63.5, 41) ccw
  line L15 (-71.5, 41) -> (-71.5, -41)
  line L16 (56.75, 6.75) -> (56.75, 16.75)
  line L17 (56.75, -6.75) -> (56.75, -16.75)
  line L18 (63, 16.75) -> (50.5, 16.75)
  line L19 (63, -16.75) -> (50.5, -16.75)
  line L20 (50.5, 16.75) -> (50.5, 29.75)
  line L21 (50.5, -16.75) -> (50.5, -29.75)
  line L22 (50.5, -29.75) -> (63, -29.75)
  line L23 (63, -29.75) -> (63, -16.75)
  line L24 (50.5, 29.75) -> (63, 29.75)
  line L25 (63, 29.75) -> (63, 16.75)
  line L26 (50.5, 25.6389) -> (50.5, 20.6389)
  line L27 (50.5, -20.8611) -> (50.5, -25.8611)
  line L28 (50.5, -25.8611) -> (63, -25.8611)
  line L29 (50.5, -20.8611) -> (63, -20.8611)
  line L30 (50.5, 20.6389) -> (63, 20.6389)
  line L31 (50.5, 25.6389) -> (63, 25.6389)
  line L32 (65, -31.75) -> (65, -14.75)
  line L33 (65, -14.75) -> (48.5, -14.75)
  line L34 (48.5, -14.75) -> (48.5, -31.75)
  line L35 (48.5, -31.75) -> (65, -31.75)
  line L36 (65, 31.75) -> (65, 14.75)
  line L37 (65, 14.75) -> (48.5, 14.75)
  line L38 (48.5, 14.75) -> (48.5, 31.75)
  line L39 (48.5, 31.75) -> (65, 31.75)
  point P0 (50.5, 23.1389)
  point P1 (50.5, -23.3611)
  dimension "d38" = 10
  dimension "d39" = 10
  dimension "d40" = 12.5
  dimension "d41" = 12.5
  dimension "d42" = 13
  dimension "d43" = 13
  dimension "d44" = 12.5
  dimension "d45" = 12.5
  dimension "d46" = 5
  dimension "d47" = 5
  dimension "d48" = 2
  dimension "d49" = -2
  constraint midpoint L1 L16.start
  constraint perpendicular L1 L16
  constraint midpoint L3 L17.start
  constraint perpendicular L3 L17
  constraint midpoint L16.end L18
  constraint perpendicular L16 L18
  constraint midpoint L17.end L19
  constraint perpendicular L17 L19
  constraint perpendicular L18 L20
  constraint perpendicular L19 L21
  constraint perpendicular L21 L22
  constraint perpendicular L20 L24
  constraint midpoint L26 P0
  constraint coincident L20 P0
  constraint perpendicular L24 L26
  constraint midpoint L27 P1
  constraint coincident L21 P1
  constraint perpendicular L3 L27
  constraint coincident L23 L28.end
  constraint perpendicular L23 L28
  constraint coincident L23 L29.end
  constraint perpendicular L23 L29
  constraint coincident L25 L30.end
  constraint perpendicular L25 L30
  constraint coincident L25 L31.end
  constraint perpendicular L25 L31
  measures "d38" distance of L16.start L16.end
  measures "d39" distance of L17.start L17.end
  measures "d40" distance of L18.start L18.end
  measures "d41" distance of L19.start L19.end
  measures "d42" distance of L18.end L20.end
  measures "d43" distance of L19.end L21.end
  measures "d44" distance of L21.end L22.end
  measures "d45" distance of L20.end L24.end
  measures "d46" distance of L26.start L26.end
  measures "d47" distance of L27.start L27.end
extrude "Extruir5" add sketch "Boceto5" along normal blind 4 contours L32 L33 L34 L35 | L36 L37 L38 L39
extrude "Extruir6" cut sketch "Boceto5" against normal blind 3 contours L18 L20 L25 L30 | L20 L24 L25 L31 | L19 L21 L23 L29 | L21 L22 L23 L28
sketch "Boceto6" plane through (0, 0, 3) normal (0, 0, 1) x (-1, 0, 0)
  line L0 (48.5, -31.75) -> (48.5, -14.75)
  line L1 (48.5, -14.75) -> (65, -14.75)
  line L2 (65, -14.75) -> (65, -31.75)
  line L3 (65, -31.75) -> (48.5, -31.75)
  line L4 (52, -6.75) -> (52, 6.75)
  line L5 (52, 6.75) -> (61.5, 6.75)
  line L6 (61.5, 6.75) -> (61.5, -6.75)
  line L7 (61.5, -6.75) -> (52, -6.75)
  line L8 (50, -10) -> (40, -10)
  line L9 (40, -10) -> (40, 10)
  line L10 (40, 10) -> (50, 10)
  line L11 (50, 10) -> (50, -10)
  line L12 (-50, -10) -> (-50, 10)
  line L13 (-50, 10) -> (-40, 10)
  line L14 (-40, 10) -> (-40, -10)
  line L15 (-40, -10) -> (-50, -10)
  circle A0 centre (62.5, 40) radius 2
  circle A1 centre (-62.5, -40) radius 2
  circle A2 centre (62.5, -40) radius 2
  circle A3 centre (-62.5, 40) radius 2
  arc A4 (-71.5, -41) -> (-63.5, -49) centre (-63.5, -41) ccw
  line L16 (-63.5, -49) -> (63.5, -49)
  arc A5 (63.5, -49) -> (71.5, -41) centre (63.5, -41) ccw
  line L17 (71.5, -41) -> (71.5, 41)
  arc A6 (71.5, 41) -> (63.5, 49) centre (63.5, 41) ccw
  line L18 (63.5, 49) -> (-63.5, 49)
  arc A7 (-63.5, 49) -> (-71.5, 41) centre (-63.5, 41) ccw
  line L19 (-71.5, 41) -> (-71.5, -41)
  line L20 (48.5, 31.75) -> (65, 31.75)
  line L21 (65, 31.75) -> (65, 14.75)
  line L22 (65, 14.75) -> (48.5, 14.75)
  line L23 (48.5, 14.75) -> (48.5, 31.75)
  line L24 (-71.5, 0) -> (-61.5, 0)
  line L25 (-61.5, -5) -> (-61.5, 5)
  circle A8 centre (-61.5, 5) radius 1.5
  circle A9 centre (-61.5, -5) radius 1.5
  dimension "d54" = 10
  dimension "d55" = 10
  dimension "d56" = 3
  dimension "d57" = 3
  constraint midpoint L19 L24.start
  constraint perpendicular L19 L24
  constraint midpoint L24.end L25
  constraint perpendicular L24 L25
  constraint coincident L25.end A8.centre
  constraint coincident L25.start A9.centre
  measures "d54" distance of L24.start L24.end
  measures "d55" distance of L25.start L25.end
  measures "d56" diameter of A8
  measures "d57" diameter of A9
extrude "Extruir7" cut sketch "Boceto6" against normal blind 3 contours A8 | A9

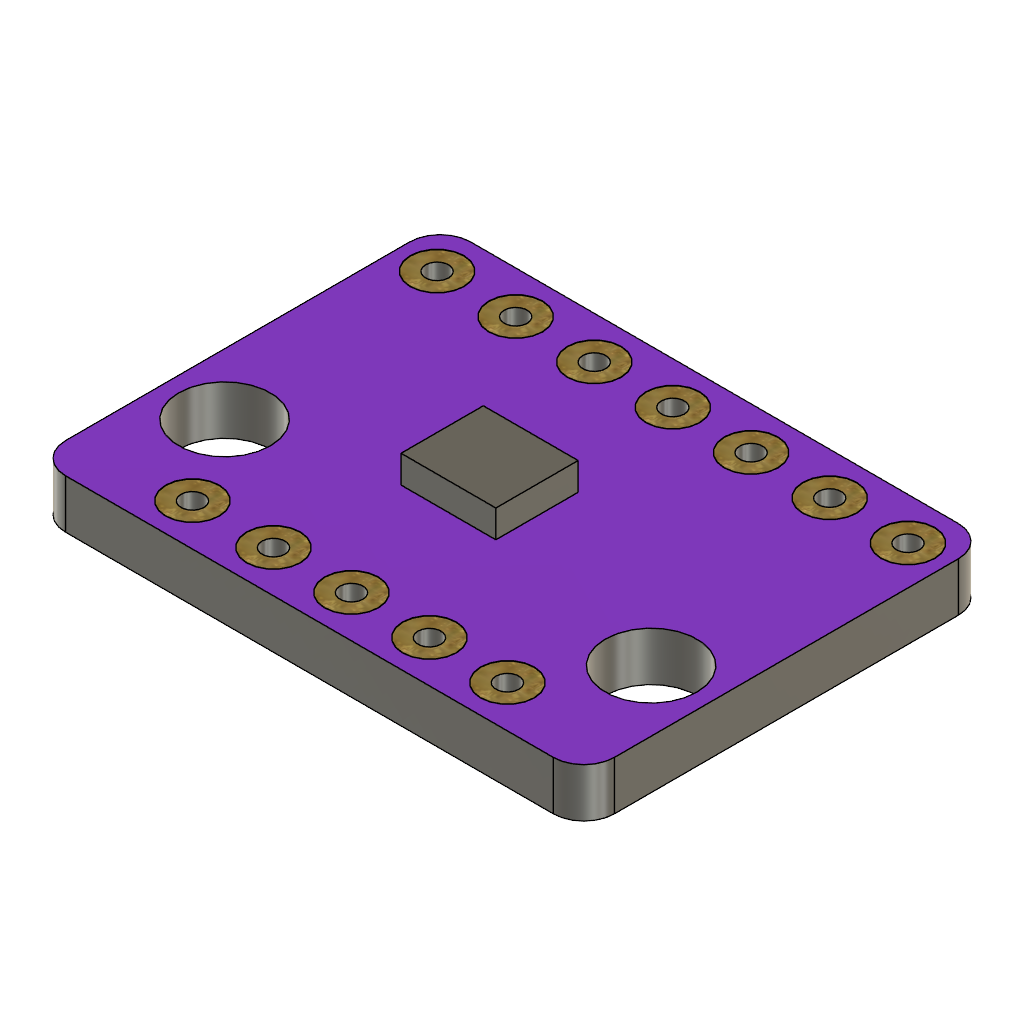
design "bmi160 v1"
Autodesk Fusion 360 part; units mm, degrees
sketch "Sketch2" plane through (0, 0, 0) normal (0, 0, 1) x (1, 0, 0)
  line L0 (-8.9478, 7.7363) -> (9.0022, 7.7363)
  line L1 (9.0022, 7.7363) -> (9.0022, -5.5137)
  line L2 (9.0022, -5.5137) -> (-8.9478, -5.5137)
  line L3 (-8.9478, -5.5137) -> (-8.9478, 7.7363)
  line L4 (-8.9478, 7.7363) -> (9.0022, -5.5137) construction
  line L5 (-8.9478, -5.5137) -> (9.0022, 7.7363) construction
  line L6 (-9.5685, 6.7363) -> (10, 6.7363) construction
  line L7 (-9.5685, 6.3613) -> (10, 6.3613) construction
  line L8 (-10.5, -4.5137) -> (10.5, -4.5137) construction
  line L9 (-10.5, -4.1387) -> (10.5, -4.1387) construction
  line L10 (8.5022, 9) -> (8.5022, -6.5) construction
  line L11 (7.0022, 9) -> (7.0022, -6.5) construction
  line L12 (-8.4478, 9.5) -> (-8.4478, -7) construction
  line L13 (-6.9478, 9.5) -> (-6.9478, -7) construction
  line L14 (-10.5, -2.8137) -> (11.6299, -2.8137) construction
  line L15 (-10.5, -1.3137) -> (11.6299, -1.3137) construction
  circle A0 centre (7.0022, -1.3137) radius 1.5
  circle A1 centre (-6.9478, -1.3137) radius 1.5
  line L16 (-8.0478, 9) -> (-8.0478, 5) construction
  line L17 (-7.6728, 9) -> (-7.6728, 5) construction
  circle A2 centre (-7.6728, 6.3613) radius 0.375
  line L18 (-5.1028, 7.3) -> (-5.1028, 4.898) construction
  circle A3 centre (-5.1028, 6.3613) radius 0.375
  circle A4 centre (-2.5328, 6.3613) radius 0.375
  circle A5 centre (0.0372, 6.3613) radius 0.375
  circle A6 centre (2.5972, 6.3613) radius 0.375
  circle A7 centre (5.1672, 6.3613) radius 0.375
  circle A8 centre (7.7272, 6.3613) radius 0.375
  circle A9 centre (-7.6728, 6.3613) radius 0.875
  line L19 (-5.5478, -3.163) -> (-5.5478, -6) construction
  line L20 (-5.1728, -3.163) -> (-5.1728, -6) construction
  circle A10 centre (-5.1728, -4.1387) radius 0.375
  line L21 (-2.1478, -3.7) -> (-2.1478, -5.9) construction
  circle A11 centre (-2.5228, -4.1387) radius 0.375
  line L22 (-2.8978, -3.7) -> (-2.8978, -5.1) construction
  line L23 (0.4022, -3.6) -> (0.4022, -5.1) construction
  circle A12 centre (0.0272, -4.1387) radius 0.375
  line L24 (-0.3478, -3.6) -> (-0.3478, -5.3) construction
  circle A13 centre (2.5772, -4.1387) radius 0.375
  circle A14 centre (5.1272, -4.1387) radius 0.375
  line L25 (2.2022, -3.6) -> (2.2022, -5.1) construction
  line L26 (4.7522, -3.7) -> (4.7522, -5.1) construction
  line L27 (2.9522, -3.8) -> (2.9522, -4.9) construction
  line L28 (5.5022, -3.7) -> (5.5022, -5.1) construction
  circle A15 centre (-5.1028, 6.3613) radius 0.875
  circle A16 centre (-2.5328, 6.3613) radius 0.875
  circle A17 centre (0.0372, 6.3613) radius 0.875
  circle A18 centre (2.5972, 6.3613) radius 0.875
  circle A19 centre (5.1672, 6.3613) radius 0.875
  circle A20 centre (7.7272, 6.3613) radius 0.875
  circle A21 centre (5.1272, -4.1387) radius 0.875
  circle A22 centre (2.5772, -4.1387) radius 0.875
  circle A23 centre (0.0272, -4.1387) radius 0.875
  circle A24 centre (-2.5228, -4.1387) radius 0.875
  circle A25 centre (-5.1728, -4.1387) radius 0.875
  line L29 (-2.2, 2.4) -> (0.9, 2.4)
  line L30 (0.9, 2.4) -> (0.9, -0.2901)
  line L31 (0.9, -0.2901) -> (-2.2, -0.2901)
  line L32 (-2.2, -0.2901) -> (-2.2, 2.4)
  dimension "d1" = 17.95
  dimension "d2" = 13.25
  dimension "d3" = 1
  dimension "d4" = 0.375
  dimension "d5" = 1
  dimension "d6" = -0.375
  dimension "d7" = 0.5
  dimension "d8" = 1.5
  dimension "d9" = 0.5
  dimension "d10" = -1.5
  dimension "d11" = 2.7
  dimension "d12" = -1.5
  dimension "d13" = 3
  dimension "d14" = 3
  dimension "d15" = 0.9
  dimension "d17" = 0.75
  dimension "d19" = 2.57
  dimension "d21" = 0.75
  dimension "d22" = 0.75
  dimension "d23" = 2.57
  dimension "d24" = 0.75
  dimension "d25" = 2.57
  dimension "d26" = 0.75
  dimension "d27" = 2.56
  dimension "d28" = 0.75
  dimension "d29" = 2.57
  dimension "d30" = 0.75
  dimension "d31" = 2.56
  dimension "d32" = 0.5
  dimension "d33" = 3.4
  dimension "d34" = -0.375
  dimension "d35" = 0.75
  dimension "d36" = 3.4
  dimension "d37" = 0.75
  dimension "d38" = 0.75
  dimension "d39" = 3.3
  dimension "d40" = 0.75
  dimension "d41" = 0.75
  dimension "d42" = 3.3
  dimension "d43" = 3.3
  dimension "d44" = 0.5
  dimension "d45" = 0.5
  dimension "d46" = 0.5
  dimension "d47" = 0.5
  dimension "d48" = 0.5
  dimension "d49" = 0.5
  dimension "d50" = 0.5
  dimension "d51" = 0.5
  dimension "d52" = 0.5
  dimension "d53" = 0.5
  dimension "d54" = 0.5
  constraint horizontal L0
  constraint vertical L1
  constraint horizontal L2
  constraint vertical L3
  constraint perpendicular L1 L6
  constraint perpendicular L3 L8
  constraint perpendicular L2 L10
  constraint perpendicular L2 L12
  constraint perpendicular L10 L14
  constraint coincident L15 A0.centre
  constraint coincident L11 A0.centre
  constraint coincident L15 A1.centre
  constraint coincident L13 A1.centre
  constraint perpendicular L7 L16
  constraint coincident L17 A2.centre
  constraint coincident L7 A2.centre
  constraint coincident L4 L18.end
  constraint perpendicular L6 L18
  constraint coincident L7 A3.centre
  constraint coincident L18 A3.centre
  constraint coincident L7 A4.centre
  constraint coincident L7 A5.centre
  constraint coincident L7 A6.centre
  constraint coincident L7 A7.centre
  constraint coincident L7 A8.centre
  constraint perpendicular L2 L19
  constraint coincident L20 A10.centre
  constraint coincident L9 A10.centre
  constraint perpendicular L2 L21
  constraint coincident L9 A11.centre
  constraint tangent L21 A11
  constraint vertical L22
  constraint tangent A11 L22
  constraint perpendicular L9 L23
  constraint coincident L9 A12.centre
  constraint tangent L23 A12
  constraint perpendicular L8 L24
  constraint tangent A12 L24
  constraint coincident L9 A13.centre
  constraint coincident L9 A14.centre
  constraint vertical L25
  constraint perpendicular L9 L26
  constraint perpendicular L9 L27
  constraint perpendicular L8 L28
  constraint tangent A14 L26
  constraint tangent A14 L28
  constraint tangent A13 L27
  constraint tangent A13 L25
  constraint horizontal L29
  constraint vertical L30
  constraint horizontal L31
  constraint vertical L32
  measures "d1" distance of L0.start L0.end
  measures "d2" distance of L0.start L2.end
  measures "d3" distance of L0 L6
  measures "d5" distance of L2 L8
  measures "d7" distance of L1 L10
  measures "d9" distance of L3 L12
  measures "d11" distance of L2 L14
  measures "d13" diameter of A0
  measures "d14" diameter of A1
  measures "d15" distance of L3 L16
  measures "d17" diameter of A2
  measures "d19" distance of A2.centre L18
  measures "d21" diameter of A3
  measures "d22" diameter of A4
  measures "d23" distance of L18 A4.centre
  measures "d24" diameter of A5
  measures "d25" distance of A4.centre A5.centre
  measures "d26" diameter of A6
  measures "d27" distance of A5.centre A6.centre
  measures "d28" diameter of A7
  measures "d29" distance of A6.centre A7.centre
  measures "d30" diameter of A8
  measures "d31" distance of A7.centre A8.centre
  measures "d33" distance of L3 L19
  measures "d35" diameter of A10
  measures "d36" distance of L19 L21
  measures "d37" diameter of A11
  measures "d38" diameter of A12
  measures "d39" distance of L22 L23
  measures "d40" diameter of A13
  measures "d41" diameter of A14
  measures "d42" distance of L24 L27
  measures "d43" distance of L25 L28
extrude "Extrude1" add sketch "Sketch2" along normal blind 1.6 contours L0 L1 L2 L3 | A9 | A15 | A16 | A17 | A18 | A19 | A20 | A21 | A22 | A23 | A24 | A25 | L29 L30 L31 L32
extrude "Extrude2" add sketch "Sketch2" along normal blind 2.5 contours L29 L30 L31 L32
fillet "Fillet1" radius 1 4 edges at (-8.9478, -5.5137, 0.8) (9.0022, -5.5137, 0.8) (9.0022, 7.7363, 0.8) (-8.9478, 7.7363, 0.8)